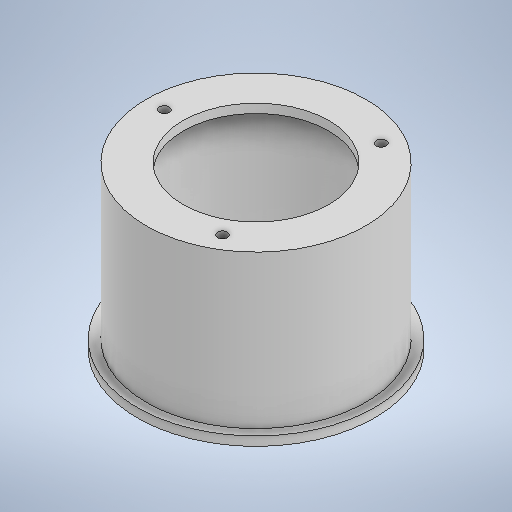
# Autodesk Inventor part: Mithril Center Cylinder
Saved by Autodesk Inventor 2026.2 (Build 302298000, 298)
## iProperties
Created: 2026-03-06
Part Number: Mithril Center Cylinder
Material: Generic
Document SubType Name: Modeling
Designer: mumin
Density: 1 g/cm^3
Appearance: Default
Author: mumin
Autodesk Inventor part; units mm, degrees
ref_plane "YZ Plane" through (0, 0, 0) normal (1, 0, 0) x (0, 1, 0)
ref_plane "XZ Plane" through (0, 0, 0) normal (0, 1, 0) x (-1, 0, 0)
ref_plane "XY Plane" through (0, 0, 0) normal (0, 0, 1) x (1, 0, 0)
sketch "Sketch1" plane through (0, 0, 0) normal (1, 0, 0) x (0, 1, 0)
  line L0 (0, 0) -> (100, 0)
  line L1 (90, -40.5) -> (85, -40.5)
  line L2 (85, -40.5) -> (85, -56)
  line L3 (85, -56) -> (0, -56)
  line L4 (0, -56) -> (0, -66)
  line L5 (0, -66) -> (5, -66)
  line L6 (5, -66) -> (5, -61)
  line L7 (5, -61) -> (90, -61)
  line L8 (90, -61) -> (90, -40.5)
  point P0 (87.5, -40.5)
  dimension "d0" = 100
  dimension "d1" = 81
  dimension "d2" = 122
  dimension "d3" = 90
  dimension "d4" = 5
  dimension "d5" = 5
  dimension "d6" = 5
  dimension "d7" = 10
  constraints: 18 end point, 7 perpendicular, 2 horizontal, 1 midpoint, 1 point on line
  measures "d0" distance of L0.start L0.end
  measures "d1" diameter of point (87.5, -40.5) L0
  measures "d2" diameter of L7 L0
  measures "d3" distance between parallel lines of L4 L8
  measures "d4" distance between parallel lines of L2 L8
  measures "d5" distance between parallel lines of L4 L6
  measures "d6" distance between parallel lines of L7 L3
  measures "d7" distance between parallel lines of L5 L3
revolve "Revolution1" add sketch "Sketch1" angle 360 about axis through (0, 0, 0) along (0, 1, 0)
sketch "Sketch2" plane through (0, 90, 0) normal (0, 1, 0) x (1, 0, 0)
  circle A0 centre (0, 0) radius 51
  point P0 (-51, 0)
  point P1 (25.5, -44.1673)
  point P2 (25.5, 44.1673)
  dimension "d9" = 102
  dimension "d12" = 360
  constraints: 1 coincident, 1 horizontal alignment, 6 other
hole "Hole1" at (-51, 90, 0) at (25.5, 90, 44.1673) at (25.5, 90, -44.1673) direction (0, -1, 0) diameter 5.5 end up to face face through (29.3624, 85, 41.2331) facing (0, -1, 0)
body "Solid1"
